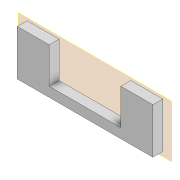
# Autodesk Inventor part: 30_XYTabel_Aliexpress_cellSTORM_chiptray_spacer
Saved by Autodesk Inventor 2022 (Build 260153000, 153)
## iProperties
Created: 2022-01-03
Part Number: 30_XYTabel_Aliexpress_cellSTORM_chiptray_spacer
Material: Generisch
Document SubType Name: Modeling
Designer: diederichbenedict
Density: 1 g/cm^3
Appearance: Vorgabe
Author: diederichbenedict
Autodesk Inventor part; units mm, degrees
ref_plane "YZ Plane" through (0, 0, 0) normal (1, 0, 0) x (0, 1, 0)
ref_plane "XZ Plane" through (0, 0, 0) normal (0, 1, 0) x (-1, 0, 0)
ref_plane "XY Plane" through (0, 0, 0) normal (0, 0, 1) x (1, 0, 0)
ref_plane "Arbeitsebene1" through (-11.4334, 18.48, -9.3955) normal (0, 0, 1) x (1, 0, 0)
sketch "Skizze1" plane through (-11.4334, 18.48, -9.3955) normal (0, 0, 1) x (1, 0, 0)
  line L0 (-38, 14.4) -> (38, 14.4) projected
  line L1 (-38, -11.4) -> (-38, 14.4) projected
  line L2 (38, -11.4) -> (-38, -11.4) projected
  line L3 (38, 14.4) -> (38, -11.4) projected
  line L4 (-37.8, 14.2) -> (37.8, 14.2)
  line L5 (37.8, 14.2) -> (37.8, -11.2)
  line L6 (37.8, -11.2) -> (-37.8, -11.2)
  line L7 (-37.8, -11.2) -> (-37.8, 14.2)
  line L8 (20, 34.2) -> (-20, 34.2)
  line L9 (-20, 34.2) -> (-20, -5.8)
  line L10 (-20, -5.8) -> (20, -5.8)
  line L11 (20, -5.8) -> (20, 34.2)
  line L12 (20, 34.2) -> (-20, -5.8) construction
  line L13 (-20, 34.2) -> (20, -5.8) construction
  point P0 (11.4334, -18.48)
  point P1 (0, 14.2)
  point P2 (-20, 14.2)
  point P3 (20, 14.2)
  point P4 (20, 14.2)
  point P5 (-20, 14.2)
  dimension "d0" = 0.2
  dimension "d1" = 20
  dimension "d2" = 40
  constraints: 20 end point, 5 midpoint, 2 parallel, 1 horizontal, 1 perpendicular, 3 other
  measures "d0" distance between parallel lines of L1 L7
  measures "d1" distance between parallel lines of L10 L4
  measures "d2" distance between parallel lines of L11 L9
extrude "Extrusion1" add sketch "Skizze1" along normal blind 5.5 contours L9 L10 L11 L4 L5 L6 L7
